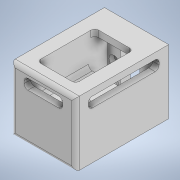
# Autodesk Inventor part: Link1r_v2
Saved by Autodesk Inventor 2022 (Build 260153000, 153)
## iProperties
Created: 2022-06-03
Part Number: Link1r_v2
Material: Generic
Document SubType Name: Modeling
Designer: Asus
Density: 1 g/cm^3
Appearance: Default
Author: Asus
Autodesk Inventor part; units mm, degrees
ref_plane "YZ Plane" through (0, 0, 0) normal (1, 0, 0) x (0, 1, 0)
ref_plane "XZ Plane" through (0, 0, 0) normal (0, 1, 0) x (-1, 0, 0)
sketch "Sketch1" plane through (0, 0, 0) normal (0, 1, 0) x (-1, 0, 0)
  line L0 (25, 22.5) -> (-25, 22.5)
  line L1 (-25, 22.5) -> (-25, -122.5)
  line L2 (-25, -122.5) -> (25, -122.5)
  line L3 (25, -122.5) -> (25, 22.5)
  circle A0 centre (0, 0) radius 3.4379
  dimension "d0" = 50
  dimension "d1" = 145
  dimension "d2" = 25
  dimension "d3" = 22.5
  dimension "d4" = 6.8759
  dimension "d5" = 0
  dimension "d6" = 0
  constraints: 8 end point, 2 parallel, 1 centre point, 1 horizontal, 1 perpendicular
  measures "d0" distance of L1.end L2.end
  measures "d1" distance of L0.end L1.end
  measures "d2" distance from line of L3 A0.centre
  measures "d3" distance from line of L0 A0.centre
  measures "d4" diameter of A0
  measures "d5" distance of point (0, 0) A0.centre
  measures "d6" distance of A0.centre point (0, 0)
extrude "Extrusion1" add sketch "Sketch1" along normal blind 5 contours L3 L2 L1 L0 | A0
sketch "Sketch2" plane through (0, 5, 0) normal (0, 1, 0) x (1, 0, 0)
  line L0 (-20, -17.5) -> (20, -17.5)
  line L1 (20, -17.5) -> (20, 117.5)
  line L2 (20, 117.5) -> (-20, 117.5)
  line L3 (-20, 117.5) -> (-20, -17.5)
  line L4 (-25, -22.5) -> (25, -22.5) projected
  line L5 (-25, 122.5) -> (-25, -22.5) projected
  line L6 (25, -22.5) -> (25, 122.5) projected
  line L7 (25, 122.5) -> (-25, 122.5) projected
  line L8 (-25, 72.5) -> (25, 72.5)
  point P0 (0, 0)
  point P1 (-20, 72.5)
  point P2 (20, 72.5)
  dimension "d9" = 5
  dimension "d10" = 5
  dimension "d11" = 5
  dimension "d12" = 5
  dimension "d13" = 50
  constraints: 10 end point, 2 parallel, 2 perpendicular, 2 point on line, 1 horizontal
  measures "d9" distance between parallel lines of L4 L0
  measures "d10" distance between parallel lines of L5 L3
  measures "d11" distance between parallel lines of L6 L1
  measures "d12" distance between parallel lines of L7 L2
  measures "d13" distance between parallel lines of L7 L8
extrude "Extrusion2" add sketch "Sketch2" along normal blind 45 contours L0 L1 L8 L6 L4 L5 L3
sketch "Sketch3" plane through (0, 50, 0) normal (0, 1, 0) x (1, 0, 0)
  line L0 (-25, -22.5) -> (25, -22.5) projected
  line L1 (25, 72.5) -> (25, 122.5) projected
  line L2 (-25, -22.5) -> (25, -22.5)
  line L3 (25, -22.5) -> (25, 72.5)
  line L4 (25, 72.5) -> (-25, 72.5)
  line L5 (-25, 72.5) -> (-25, -22.5)
  point P0 (0, 0)
  constraints: 8 end point, 2 parallel, 1 horizontal, 1 perpendicular
extrude "Extrusion3" add sketch "Sketch3" against normal blind 5
sketch "Sketch4" plane through (20, 5, 17.5) normal (0, 0, -1) x (-1, 0, 0)
  line L0 (0, 0) -> (0, 40) projected
  line L1 (40, 0) -> (40, 40) projected
  line L2 (0, 20) -> (40, 20)
  line L3 (40, 20) -> (40, 0)
  line L4 (40, 0) -> (0, 0)
  line L5 (0, 0) -> (0, 20)
  point P0 (20, -5)
  dimension "d18" = 20
  constraints: 8 end point, 2 parallel, 1 horizontal, 1 midpoint, 1 perpendicular
  measures "d18" distance between parallel lines of L4 L2
extrude "Extrusion4" add sketch "Sketch4" along normal blind 45
sketch "Sketch5" plane through (0, 0, 0) normal (0, -1, 0) x (1, 0, 0)
  circle A0 centre (0, 0) radius 9.5
  dimension "d21" = 19
  constraints: 1 centre point, 1 coincident
  measures "d21" diameter of A0
extrude "Extrusion5" cut sketch "Sketch5" against normal blind 12
sketch "Sketch6" plane through (0, 0, 0) normal (0, -1, 0) x (1, 0, 0)
  circle A0 centre (0, 0) radius 11.5
  dimension "d24" = 23
  constraints: 1 centre point, 1 coincident
  measures "d24" diameter of A0
extrude "Extrusion6" cut sketch "Sketch6" against normal blind 6.5
sketch "Sketch7" plane through (0, 12, 0) normal (0, -1, 0) x (1, 0, 0)
  circle A0 centre (0, 0) radius 6.2
  line L0 (0, 6.7252) -> (0, 0)
  line L1 (0, 0) -> (-6.727, -3.8838)
  line L2 (0, 0) -> (6.6601, -3.8452)
  circle A1 centre (0, 6.2) radius 1.45
  circle A2 centre (-5.3694, -3.1) radius 1.45
  circle A3 centre (5.3694, -3.1) radius 1.45
  dimension "d27" = 12.4
  dimension "d28" = 120
  dimension "d29" = 120
  dimension "d30" = 2.9
  dimension "d31" = 2.9
  dimension "d32" = 2.9
  constraints: 6 end point, 4 centre point, 3 point on circle, 3 point on line, 1 coincident, 1 vertical
  measures "d27" diameter of A0
  measures "d28" angle of L1 L0
  measures "d29" angle of L2 L1
  measures "d30" diameter of A1
  measures "d31" diameter of A3
  measures "d32" diameter of A2
extrude "Extrusion7" cut sketch "Sketch7" against normal blind 15 contours A1 L0 A0 | A0 A1 | A3 L2 A0 | A0 L2 A3 | L0 A1 A0 | L2 A3 A0 | A0 A3 L2 | A2 L1 A0 | A0 L1 A2 | A2 A0 L1 | A2 L1 A0
sketch "Sketch8" plane through (-20, 25, 17.5) normal (0, 1, 0) x (1, 0, 0)
  circle A0 centre (14.6306, 20.6) radius 1.45 projected
  circle A1 centre (14.6306, 20.6) radius 4
  circle A2 centre (20, 11.3) radius 1.45 projected
  circle A3 centre (20, 11.3) radius 4
  circle A4 centre (25.3694, 20.8298) radius 4
  point P0 (20, 17.5)
  dimension "d35" = 8
  dimension "d36" = 8
  dimension "d37" = 8
  constraints: 3 centre point, 2 coincident
  measures "d35" diameter of A4
  measures "d36" diameter of A3
  measures "d37" diameter of A1
extrude "Extrusion8" cut sketch "Sketch8" against normal blind 7
sketch "Sketch10" plane through (-20, 5, -72.5) normal (1, 0, 0) x (0, 0, -1)
  line L0 (-45, 20) -> (-45, 0) projected
  line L1 (-45, 0) -> (50, 0)
  line L2 (50, 0) -> (50, 45)
  line L3 (50, 45) -> (-45, 45)
  line L4 (-45, 45) -> (-45, 0)
  point P0 (-72.5, -5)
  dimension "d44" = 45
  dimension "d45" = 95
  constraints: 8 end point, 2 parallel, 1 horizontal, 1 perpendicular
  measures "d44" distance of L1.end L2.end
  measures "d45" distance of L2.end L3.end
extrude "Extrusion9" add sketch "Sketch10" against normal blind 5
sketch "Sketch11" plane through (-20, 5, -122.5) normal (1, 0, 0) x (0, 0, -1)
  line L0 (-140, 20) -> (-95, 20) projected
  line L1 (-140, 40) -> (-140, 20)
  line L2 (-140, 20) -> (-95, 20)
  line L3 (-95, 20) -> (-95, 0.1891)
  line L4 (0, 0) -> (-95, 0) projected
  line L5 (-95, 0.1891) -> (-95, 0)
  line L6 (-95, 0) -> (0, 0)
  line L7 (0, 0) -> (0, 45) projected
  line L8 (0, 0) -> (0, 45)
  line L9 (0, 45) -> (-50, 45)
  line L10 (-50, 40) -> (-50, 45) projected
  line L11 (-50, 45) -> (-50, 40)
  line L12 (-50, 40) -> (-140, 40)
  point P0 (-122.5, -5)
  point P1 (-50, 45)
  constraints: 18 end point, 5 perpendicular, 3 collinear, 1 vertical
extrude "Extrusion10" add sketch "Sketch11" along normal blind 5
sketch "Sketch12" plane through (-15, 5, -122.5) normal (1, 0, 0) x (0, 0, -1)
  circle A0 centre (-22.5, 20) radius 6.5
  circle A1 centre (50.1316, 17.215) radius 18.4
  circle A2 centre (57.8816, 30.6384) radius 1.5
  circle A3 centre (57.8816, 30.6384) radius 1.5
  circle A4 centre (65.6316, 17.215) radius 1.5
  circle A5 centre (65.6316, 17.215) radius 1.5
  circle A6 centre (57.8816, 3.7916) radius 1.5
  circle A7 centre (57.8816, 3.7916) radius 1.5
  circle A8 centre (42.3816, 3.7916) radius 1.5
  circle A9 centre (42.3816, 3.7916) radius 1.5
  circle A10 centre (34.6316, 17.215) radius 1.5
  circle A11 centre (34.6316, 17.215) radius 1.5
  circle A12 centre (42.3816, 30.6384) radius 1.5
  circle A13 centre (42.3816, 30.6384) radius 1.5
  circle A14 centre (50.1316, 17.215) radius 15.5
  circle A15 centre (50.1316, 17.215) radius 18.4
  line L0 (57.8816, 30.6384) -> (50.1316, 17.215)
  line L1 (50.1316, 17.215) -> (65.6316, 17.215)
  line L2 (42.3816, 3.7916) -> (50.1316, 17.215)
  line L3 (50.1316, 17.215) -> (34.6316, 17.215)
  line L4 (42.3816, 30.6384) -> (50.1316, 17.215)
  line L5 (57.8816, 3.7916) -> (50.1316, 17.215)
  circle A16 centre (50.1316, 10.215) radius 6
  circle A17 centre (50.1316, 10.215) radius 6
  circle A18 centre (-22.5, 27) radius 15.5
  line L6 (0, 0) -> (0, 45) projected
  line L7 (0, 45) -> (-50, 45) projected
  line L8 (-22.5, 27) -> (-4.9973, 27)
  line L9 (-22.5, 27) -> (-39.7636, 27)
  line L10 (-22.5, 27) -> (-13.3528, 42.8433)
  line L11 (-22.5, 27) -> (-30.25, 40.4234)
  line L12 (-22.5, 27) -> (-30.25, 13.5766)
  line L13 (-22.5, 27) -> (-14.75, 13.5766)
  circle A19 centre (-14.75, 40.4234) radius 1.5
  circle A20 centre (-30.25, 40.4234) radius 1.5
  circle A21 centre (-7, 27) radius 1.5
  circle A22 centre (-38, 27) radius 1.5
  circle A23 centre (-30.25, 13.5766) radius 1.5
  circle A24 centre (-14.75, 13.5766) radius 1.5
  point P0 (-122.5, -5)
  dimension "d60" = 31
  dimension "d52" = 13
  dimension "d53" = 36.8
  dimension "d54" = 3
  dimension "d55" = 3
  dimension "d56" = 3
  dimension "d57" = 3
  dimension "d58" = 3
  dimension "d59" = 3
  dimension "d61" = 7
  dimension "d62" = 60
  dimension "d63" = 60
  dimension "d64" = 15.5
  dimension "d65" = 12
  dimension "d66" = 31
  dimension "d67" = 7
  dimension "d68" = 22.5
  dimension "d69" = 18
  dimension "d70" = 25
  dimension "d71" = 60
  dimension "d72" = 60
  dimension "d73" = 60
  dimension "d74" = 3
  dimension "d75" = 3
  dimension "d76" = 3
  dimension "d77" = 3
  dimension "d78" = 3
  dimension "d79" = 3
  constraints: 24 centre point, 24 end point, 12 coincident, 6 point on circle, 5 point on line, 3 collinear, 1 horizontal, 1 horizontal alignment, 1 perpendicular, 2 other
  measures "d52" diameter of A0
  measures "d53" diameter of A1
  measures "d54" diameter of A2
  measures "d55" diameter of A4
  measures "d56" diameter of A7
  measures "d57" diameter of A8
  measures "d58" diameter of A10
  measures "d59" diameter of A13
  measures "d61" distance of point (50.132, 17.215) A16.centre
  measures "d62" angle of L1 L0
  measures "d63" angle of L4 L3
  measures "d64" distance of L0.start L0.end
  measures "d65" diameter of A16
  measures "d66" diameter of A18
  measures "d67" distance of L8.start A0.centre
  measures "d68" distance from line of L6 L8.start
  measures "d69" distance from line of L7 L8.start
  measures "d70" distance from line of L7 A0.centre
  measures "d71" angle of L8 L10
  measures "d72" angle of L9 L11
  measures "d73" angle of L9 L12
  measures "d74" diameter of A19
  measures "d75" diameter of A20
  measures "d76" diameter of A22
  measures "d77" diameter of A23
  measures "d78" diameter of A24
  measures "d79" diameter of A21
extrude "Extrusion11" cut sketch "Sketch12" against normal blind 10 contours A0 L13 | L13 A0 L12 | L12 A0 | A24 A18 L13 | L13 A18 A24 | A21 A18 L8 | L8 A18 A21 | A22 A18 L9 | L9 A18 A22 | A19 A18 L10 | L10 A18 A19 | A20 A18 L11 | L11 A18 A20 | A23 A18 L12 | L12 A18 A23 | A18 A24 | L8 A21 A18 | A18 A21 L8 | L9 A22 A18 | A18 A22 L9 | L10 A19 A18 | A18 A19 L10 | A18 A20 | A18 A23 picked at (-20.282, 19.0179)
sketch "Sketch13" plane through (0, 50, 0) normal (0, 1, 0) x (1, 0, 0)
  line L0 (-15, 27.5) -> (-15, -17.5) projected
  line L1 (20, -17.5) -> (20, 72.5) projected
  line L2 (-15, -17.5) -> (20, -17.5)
  line L3 (20, -17.5) -> (20, 27.5)
  line L4 (20, 27.5) -> (-15, 27.5)
  line L5 (-15, 27.5) -> (-15, -17.5)
  line L6 (-15, -17.5) -> (15, -17.5)
  line L7 (15, -17.5) -> (15, 27.5)
  line L8 (15, 27.5) -> (-15, 27.5)
  line L9 (-15, 27.5) -> (-15, -17.5)
  line L10 (-17.6229, -12.5) -> (23.226, -12.5)
  line L11 (25, -22.5) -> (25, 122.5) projected
  line L12 (-25, -22.5) -> (25, -22.5) projected
  point P0 (0, 0)
  point P1 (-15, 27.5)
  point P2 (-15, -12.5)
  point P3 (15, -12.5)
  dimension "d82" = 45
  dimension "d83" = 30
  dimension "d100" = 10
  constraints: 18 end point, 4 parallel, 3 perpendicular, 2 horizontal, 1 midpoint, 1 point on line
  measures "d82" distance between parallel lines of L2 L4
  measures "d83" distance between parallel lines of L0 L7
  measures "d100" distance between parallel lines of L12 L10
extrude "Extrusion12" cut sketch "Sketch13" against normal blind 10 contours L4 L7 L10 L0
sketch "Sketch14" plane through (25, 0, 22.5) normal (1, 0, 0) x (0, 0, -1)
  line L0 (145, 5) -> (50, 5) projected
  line L1 (95, 5) -> (95, 50) projected
  line L2 (10, 45) -> (85, 45)
  line L3 (85, 45) -> (85, 5)
  line L4 (85, 5) -> (10, 5)
  line L5 (10, 5) -> (10, 45)
  line L6 (0, 0) -> (0, 50) projected
  line L7 (0, 50) -> (95, 50) projected
  line L8 (0, 0) -> (145, 0) projected
  line L9 (10, 37) -> (90.8755, 37)
  line L10 (90.8755, 29) -> (3.3121, 29)
  line L11 (50, 25) -> (5, 25) projected
  line L12 (5, 21) -> (92.1289, 21)
  line L13 (3.3121, 13) -> (95, 13)
  line L14 (50, 5) -> (50, 25) projected
  line L15 (50, 5) -> (50, 25)
  line L16 (50, 25) -> (10, 25)
  line L17 (50, 25) -> (5, 25) projected
  line L18 (65, 47.5096) -> (65, 32.8574)
  point P0 (22.5, 0)
  point P1 (5, 45)
  point P2 (3.3121, 29)
  point P3 (85, 13)
  point P4 (10, 13)
  point P5 (85, 5)
  point P6 (10, 21)
  point P7 (85, 21)
  point P8 (85, 29)
  point P9 (10, 29)
  point P10 (85, 37)
  point P11 (50, 21)
  point P12 (10, 25)
  point P13 (50, 13)
  point P14 (65, 37)
  point P15 (65, 45)
  dimension "d87" = 10
  dimension "d88" = 10
  dimension "d89" = 5
  dimension "d90" = 5
  dimension "d91" = 8
  dimension "d92" = 8
  dimension "d93" = 8
  dimension "d94" = 8
  dimension "d162" = 30
  constraints: 20 end point, 5 horizontal, 3 point on line, 2 parallel, 1 collinear, 1 midpoint, 1 perpendicular, 1 vertical, 3 other
  measures "d87" distance between parallel lines of L3 L1
  measures "d88" distance between parallel lines of L6 L5
  measures "d89" distance between parallel lines of L7 L2
  measures "d90" distance between parallel lines of L8 L4
  measures "d91" distance between parallel lines of L2 L9
  measures "d94" distance between parallel lines of L12 L13
  measures "d162" distance between parallel lines of L18 L1
extrude "Extrusion13" cut sketch "Sketch14" against normal blind 5 contours L9 L5 L2 L18
fillet "Fillet1" radius 3 6 edges at (-15, 47.5, -72.5) (-15, 25, -5) (2.5, 25, 17.5) (20, 35, 17.5) (-15, 47.5, -27.5) (15, 47.5, -27.5)
fillet "Fillet2" radius 3 4 edges at (22.5, 45, 12.5) (22.5, 37, 12.5) (22.5, 37, -42.5) (22.5, 45, -42.5)
fillet "Fillet3" radius 3 4 edges at (25, 25, 22.5) (0, 0, 22.5) (-25, 25, 22.5) (0, 50, 22.5)
fillet "Fillet4" radius 3 2 edges at (-15, 47.5, 12.5) (15, 47.5, 12.5)
sketch "Sketch15" plane through (20, 5, -27.5) normal (0, 0, -1) x (-1, 0, 0)
  circle A0 centre (20, 3.75) radius 1.95
  line L0 (45, -5) -> (45, 45) projected
  line L1 (-5, -5) -> (45, -5) projected
  point P0 (20, -5)
  dimension "d102" = 25
  dimension "d103" = 8.75
  dimension "d107" = 3.9
  constraints: 1 centre point
  measures "d102" distance from line of L0 A0.centre
  measures "d103" distance from line of L1 A0.centre
  measures "d107" diameter of A0
extrude "Extrusion14" cut sketch "Sketch15" against normal blind 20
sketch "Sketch16" plane through (20, 5, -27.5) normal (0, 0, -1) x (-1, 0, 0)
  circle A0 centre (20, 3.75) radius 1.95 projected
  circle A1 centre (20, 3.75) radius 4
  point P0 (20, -5)
  dimension "d106" = 8
  constraints: 1 centre point, 1 coincident
  measures "d106" diameter of A1
extrude "Extrusion15" cut sketch "Sketch16" against normal blind 8
sketch "Sketch17" plane through (0, 5, 0) normal (0, 1, 0) x (1, 0, 0)
  line L0 (20, 72.5) -> (25, 72.5) projected
  line L1 (-15, 122.5) -> (-15, 75.5) projected
  line L2 (25, 72.5) -> (-15, 72.5)
  line L3 (-15, 72.5) -> (-15, 122.5)
  line L4 (-15, 122.5) -> (25, 122.5)
  line L5 (25, 122.5) -> (25, 72.5)
  point P0 (0, 0)
  constraints: 8 end point, 2 parallel, 1 horizontal, 1 perpendicular
extrude "Extrusion16" cut sketch "Sketch17" against normal blind 8
fillet "Fillet5" radius 3 1 edges at (-15, 2.5, -72.5)
fillet "Fillet6" radius 3 2 edges at (-20, 50, -122.5) (-20, 0, -122.5)
sketch "Sketch18" plane through (25, 0, -72.5) normal (1, 0, 0) x (0, 0, -1)
  line L0 (-92, 50) -> (0, 50) projected
  line L1 (-92, 0) -> (0, 0) projected
  line L2 (-95, 50) -> (-22.5, 50)
  line L3 (-22.5, 50) -> (-22.5, 0)
  line L4 (-22.5, 0) -> (-95, 0)
  line L5 (-95, 0) -> (-95, 50)
  line L6 (50, 47) -> (50, 3) projected
  line L7 (-95, 47) -> (-95, 3) projected
  line L8 (-22.5, 50) -> (50, 50)
  line L9 (50, 50) -> (50, 0)
  line L10 (50, 0) -> (-22.5, 0)
  line L11 (-22.5, 0) -> (-22.5, 50)
  point P0 (-72.5, 0)
  point P1 (50, 3)
  dimension "d114" = 72.5
  dimension "d115" = 0
  constraints: 16 end point, 4 parallel, 3 point on line, 2 horizontal, 2 perpendicular
  measures "d114" distance between parallel lines of L6 L3
  measures "d115" distance between parallel lines of L7 L5
ref_plane "Work Plane1" through (-22, 47, -50) normal (0, 0, 1) x (1, 0, 0)
sketch "Sketch19" plane through (-22, 47, -50) normal (0, 0, 1) x (1, 0, 0)
  line L0 (42, -2) -> (42, -5) projected
  line L1 (42, -2) -> (32, -2)
  line L2 (32, -2) -> (32, -12)
  line L3 (32, -12) -> (42, -12)
  line L4 (42, -12) -> (42, -2)
  line L5 (7, -2) -> (10, -2) projected
  line L6 (7, -2) -> (17, -2)
  line L7 (17, -2) -> (17, -12)
  line L8 (17, -12) -> (7, -12)
  line L9 (7, -12) -> (7, -2)
  line L10 (7, -42) -> (20.6081, -42) projected
  line L11 (7, -42) -> (17, -42)
  line L12 (17, -42) -> (17, -32)
  line L13 (17, -32) -> (7, -32)
  line L14 (7, -32) -> (7, -42)
  line L15 (42, -42) -> (42, -22) projected
  line L16 (42, -42) -> (32, -42)
  line L17 (32, -42) -> (32, -32)
  line L18 (32, -32) -> (42, -32)
  line L19 (42, -32) -> (42, -42)
  line L20 (17, -12) -> (32, -12)
  line L21 (32, -12) -> (32, -2)
  line L22 (32, -2) -> (17, -2)
  line L23 (17, -2) -> (17, -12)
  line L24 (32, -12) -> (42, -12)
  line L25 (42, -12) -> (42, -32)
  line L26 (42, -32) -> (32, -32)
  line L27 (32, -32) -> (32, -12)
  line L28 (17, -12) -> (7, -12)
  line L29 (7, -12) -> (7, -32)
  line L30 (7, -32) -> (17, -32)
  line L31 (17, -32) -> (17, -12)
  point P0 (22, -47)
  point P1 (42, -5)
  point P2 (10, -2)
  point P3 (32, -12)
  point P4 (32, -12)
  point P5 (32, -12)
  point P6 (32, -12)
  point P7 (42, -12)
  point P8 (7, -12)
  point P9 (17, -2)
  dimension "d117" = 10
  dimension "d118" = 10
  dimension "d119" = 10
  dimension "d120" = 10
  dimension "d121" = 10
  dimension "d122" = 10
  dimension "d123" = 10
  constraints: 56 end point, 14 parallel, 7 horizontal, 7 perpendicular, 1 point on line
  measures "d117" distance of L2.end L3.end
  measures "d118" distance of L1.end L2.end
  measures "d119" distance of L7.end L8.end
  measures "d120" distance of L12.end L13.end
  measures "d121" distance of L11.end L12.end
  measures "d122" distance of L17.end L18.end
  measures "d123" distance of L16.end L17.end
extrude "Extrusion17" add sketch "Sketch19" along normal mid plane 15
sketch "Sketch20" plane through (-22, 47, -57.5) normal (0, 0, -1) x (-1, 0, 0)
  circle A0 centre (-12, -37) radius 1.95
  circle A1 centre (-37, -37) radius 1.95
  circle A2 centre (-37, -7) radius 1.95
  circle A3 centre (-12, -7) radius 1.95
  circle A4 centre (-12, -22) radius 1.95
  circle A5 centre (-37, -22) radius 1.95
  line L0 (-7, 0) -> (-7, -44) projected
  line L1 (-42, -42) -> (-10, -42) projected
  line L2 (-10, -2) -> (-42, -2) projected
  line L3 (-42, -42) -> (-42, -2) projected
  circle A6 centre (-24.5, -7) radius 1.95
  point P0 (-22, -47)
  dimension "d126" = 5
  dimension "d127" = 5
  dimension "d128" = 3.9
  dimension "d129" = 5
  dimension "d130" = 5
  dimension "d131" = 3.9
  dimension "d132" = 5
  dimension "d133" = 5
  dimension "d134" = 3.9
  dimension "d135" = 5
  dimension "d136" = 5
  dimension "d137" = 3.9
  dimension "d138" = 15
  dimension "d139" = 5
  dimension "d140" = 3.9
  dimension "d141" = 15
  dimension "d142" = 5
  dimension "d143" = 3.9
  dimension "d158" = 3.9
  dimension "d159" = 5
  dimension "d160" = 12.5
  constraints: 7 centre point
  measures "d126" distance from line of L0 A0.centre
  measures "d127" distance from line of L1 A0.centre
  measures "d128" diameter of A0
  measures "d129" distance from line of L0 A3.centre
  measures "d130" distance from line of L2 A3.centre
  measures "d131" diameter of A3
  measures "d132" distance from line of L2 A2.centre
  measures "d133" distance from line of L3 A2.centre
  measures "d134" diameter of A2
  measures "d135" distance from line of L1 A1.centre
  measures "d136" distance from line of L3 A1.centre
  measures "d137" diameter of A1
  measures "d138" distance of A1.centre A5.centre
  measures "d139" distance from line of L3 A5.centre
  measures "d140" diameter of A5
  measures "d141" distance of A0.centre A4.centre
  measures "d142" distance from line of L0 A4.centre
  measures "d143" diameter of A4
  measures "d158" diameter of A6
  measures "d159" distance from line of L2 A6.centre
  measures "d160" distance of A3.centre A6.centre
extrude "Extrusion18" cut sketch "Sketch20" against normal blind 15
sketch "Sketch21" plane through (-22, 47, -42.5) normal (0, 0, 1) x (1, 0, 0)
  circle A0 centre (12, -22) radius 1.95 projected
  circle A1 centre (12, -22) radius 4
  circle A2 centre (12, -7) radius 1.95 projected
  circle A3 centre (12, -7) radius 4
  circle A4 centre (37, -22) radius 1.95 projected
  circle A5 centre (37, -22) radius 4
  circle A6 centre (37, -7) radius 1.95 projected
  circle A7 centre (37, -7) radius 4
  circle A8 centre (12, -37) radius 1.95 projected
  circle A9 centre (12, -37) radius 4
  circle A10 centre (37, -37) radius 1.95 projected
  circle A11 centre (37, -37) radius 4
  circle A12 centre (24.5, -7) radius 1.95 projected
  circle A13 centre (24.5, -7) radius 4
  point P0 (22, -47)
  dimension "d150" = 8
  dimension "d151" = 8
  dimension "d152" = 8
  dimension "d153" = 8
  dimension "d154" = 8
  dimension "d155" = 8
  dimension "d161" = 8
  constraints: 7 centre point, 7 coincident
  measures "d150" diameter of A1
  measures "d151" diameter of A3
  measures "d152" diameter of A5
  measures "d153" diameter of A7
  measures "d154" diameter of A9
  measures "d155" diameter of A11
  measures "d161" diameter of A13
sketch "Sketch22" plane through (0, 50, 0) normal (0, 1, 0) x (1, 0, 0)
  line L0 (-15, -9.5) -> (-15, 24.5) projected
  line L1 (-15, 24.5) -> (15, 24.5)
  line L2 (15, 24.5) -> (15, 32.5)
  line L3 (15, 32.5) -> (-15, 32.5)
  line L4 (-15, 32.5) -> (-15, 24.5)
  line L5 (-15, 42.5) -> (20, 42.5) projected
  point P0 (0, 0)
  point P1 (25, 42.5)
  dimension "d146" = 10
  constraints: 8 end point, 2 parallel, 1 horizontal, 1 perpendicular
  measures "d146" distance between parallel lines of L5 L3
extrude "Extrusion19" cut sketch "Sketch22" against normal blind 10
fillet "Fillet7" radius 3 2 edges at (-15, 47.5, -32.5) (15, 47.5, -32.5)
extrude "Extrusion20" cut sketch "Sketch21" against normal blind 4
sketch "Sketch23" plane through (-22, 47, 22.5) normal (0, 0, 1) x (1, 0, 0)
  line L0 (7, -19) -> (7, -2) projected
  line L1 (7, -2) -> (37, -2)
  line L2 (37, -2) -> (37, -10)
  line L3 (37, -10) -> (7, -10)
  line L4 (7, -10) -> (7, -2)
  line L5 (47, -47) -> (47, 3) projected
  line L6 (47, 3) -> (-3, 3) projected
  point P0 (22, -47)
  point P1 (7, -10)
  dimension "d163" = 10
  dimension "d164" = 8
  dimension "d165" = 5
  constraints: 8 end point, 2 parallel, 1 horizontal, 1 perpendicular, 1 point on line
  measures "d163" distance between parallel lines of L5 L2
  measures "d164" distance between parallel lines of L3 L1
  measures "d165" distance between parallel lines of L6 L1
extrude "Extrusion21" cut sketch "Sketch23" against normal blind 5
fillet "Fillet8" radius 3 4 edges at (15, 45, 20) (15, 37, 20) (-15, 45, 16) (-15, 37, 20)
extrude "Extrusion22" cut sketch "Sketch18" against normal blind 50 contours L0 L8 L9 L6 L10 L1 L3
body "Solid1"
